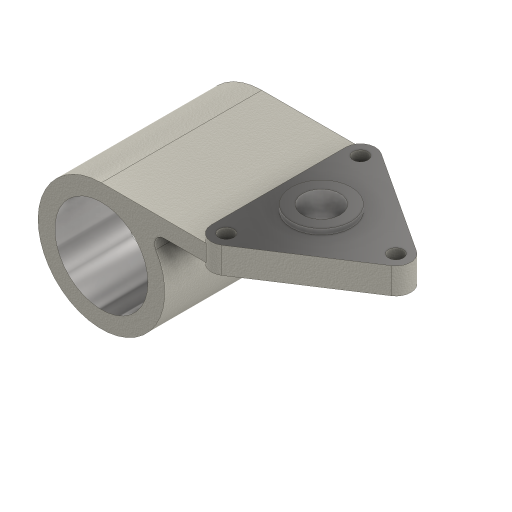
# Autodesk Inventor part: Part033.Pivoting connection
Saved by Autodesk Inventor 2023.2 (Build 272271030, 271C)
## iProperties
Created: 2023-11-14
Part Number: Part033.Pivoting connection
Material: Steel, Carbon
Document SubType Name: Modeling
Designer: User
Mass: 1782.47 g
Surface Area: 537.546 cm^2
Volume: 227.066 cm^3
Density: 7.85 g/cm^3
Appearance: Steel - Cast
Author: User
Autodesk Inventor part; units mm, degrees
note: some values were not read from the file. Chosen so that the rebuilt part matches the saved one: direction of "Hole3".
ref_plane "YZ Plane" through (0, 0, 0) normal (1, 0, 0) x (0, 1, 0)
sketch "Sketch1" plane through (0, 0, 0) normal (0, 0, 1) x (1, 0, 0)
  circle A0 centre (0, 0) radius 25
  arc A1 (0, 34) -> (23.0434, 25) centre (0, 0) ccw
  line L0 (0, 34) -> (60, 34)
  line L1 (60, 34) -> (60, 25)
  line L2 (60, 25) -> (23.0434, 25)
  arc A2 (23.0434, 25) -> (0, 34) centre (0, 0) ccw construction
  dimension "d1" = 68
  dimension "d2" = 50
  dimension "d3" = 9
  dimension "d4" = 60
  constraints: 6 end point, 4 point on circle, 3 centre point, 2 coincident, 2 perpendicular, 1 horizontal, 1 tangent
  measures "d1" diameter of A1
  measures "d2" diameter of A0
  measures "d3" distance between parallel lines of L2 L0
  measures "d4" distance from line of point (0, 0) L1
extrude "Extrusion1" add sketch "Sketch1" along normal mid plane 86
ref_plane "Work Plane1" through (0, 37, 43) normal (0, 1, 0) x (1, 0, 0)
sketch "Sketch2" plane through (0, 37, 43) normal (0, 1, 0) x (1, 0, 0)
  line L0 (60, 79) -> (115, 43) construction
  line L1 (115, 43) -> (60, 7) construction
  line L2 (60, 7) -> (60, 79) construction
  line L3 (60, 86) -> (60, 0) projected
  line L4 (119.3813, 49.6936) -> (64.3813, 85.6936)
  line L5 (52, 79) -> (52, 7)
  line L6 (64.3813, 0.3064) -> (119.3813, 36.3064)
  arc A0 (64.3813, 85.6936) -> (52, 79) centre (60, 79) ccw
  arc A1 (52, 7) -> (64.3813, 0.3064) centre (60, 7) ccw
  arc A2 (119.3813, 36.3064) -> (119.3813, 49.6936) centre (115, 43) ccw
  point P0 (0, 43)
  dimension "d8" = 55
  dimension "d9" = 72
  dimension "d10" = 8
  dimension "d11" = 8
  constraints: 12 end point, 6 point on circle, 6 tangent, 3 centre point, 2 equal radius, 1 collinear, 1 equal length, 1 horizontal alignment, 1 vertical, 2 other
  measures "d8" distance from line of L0.end L2
  measures "d9" distance of L1.end L0.start
  measures "d10" distance between parallel lines of L0 L4
  measures "d11" radius of A0
extrude "Extrusion2" add sketch "Sketch2" against normal blind 14
sketch "Sketch3" plane through (0, 37, 43) normal (0, 1, 0) x (1, 0, 0)
  arc A0 (64.3813, 85.6936) -> (52, 79) centre (60, 79) ccw projected
  arc A1 (52, 7) -> (64.3813, 0.3064) centre (60, 7) ccw projected
  arc A2 (119.3813, 36.3064) -> (119.3813, 49.6936) centre (115, 43) ccw projected
  point P0 (0, 43)
hole "Hole1" at (60, 37, 36) at (60, 37, -36) at (115, 37, 0) direction (0, -1, 0) diameter 8 end through all
sketch "Sketch4" plane through (0, 37, 43) normal (0, 1, 0) x (1, 0, 0)
  circle A0 centre (115, 43) radius 4 projected
  circle A1 centre (75, 43) radius 16
  point P0 (0, 43)
  dimension "d21" = 32
  dimension "d22" = 40
  constraints: 1 centre point, 1 horizontal alignment
  measures "d21" diameter of A1
  measures "d22" distance of A0.centre A1.centre
extrude "Extrusion3" add sketch "Sketch4" along normal blind 3 contours A1
sketch "Sketch5" plane through (75, 40, 0) normal (0, 1, 0) x (1, 0, 0)
  circle A0 centre (0, 0) radius 16 projected
  point P0 (-75, 0)
hole "Hole2" at (75, 40, 0) direction (0, -1, 0) diameter 20 end through all
ref_plane "Work Plane3" through (-31.8198, -31.8198, 0) normal (0.7071068, 0.7071068, 0) x (0, 0, 1)
ref_plane "Work Plane2" through (0, 0, 0) normal (0.7071068, 0.7071068, 0) x (0, 0, 1)
sketch "Sketch6" plane through (-31.8198, -31.8198, 0) normal (0.7071068, 0.7071068, 0) x (0, 0, 1)
  circle A0 centre (0, 0) radius 16
  dimension "d34" = 32
  constraints: 1 centre point, 1 coincident
  measures "d34" diameter of A0
extrude "Extrusion4" add sketch "Sketch6" along normal up to next
sketch "Sketch7" plane through (-31.8198, -31.8198, 0) normal (-0.7071068, -0.7071068, 0) x (-0.7071068, 0.7071068, 0)
  circle A0 centre (0, 0) radius 16 projected
hole "Hole3" at (-31.8198, -31.8198, 0) direction (0.7071068, 0.7071068, 0) diameter 16.376 end up to surface thread size "M18x1.5" class "6H" standard "ISO Metric profile"
fillet "Fillet1" radius 5 1 edges at (23.0434, 25, 0)
body "Solid1"
